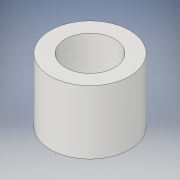
# Autodesk Inventor part: Spacer (Nylon), .313''OD, 0.25''
Saved by Autodesk Inventor 2018 (Build 220112000, 112)
## iProperties
Created: 2018-06-13
Part Number: Spacer (Nylon), .313''OD, 0.25''
Material: ABS Plastic
Document SubType Name: Modeling
Designer: s2sid
Density: 1.06 g/cm^3
Appearance: Smooth - White
Author: s2sid
Autodesk Inventor part; units mm, degrees
ref_plane "YZ Plane" through (0, 0, 0) normal (1, 0, 0) x (0, 1, 0)
ref_plane "XZ Plane" through (0, 0, 0) normal (0, 1, 0) x (-1, 0, 0)
ref_plane "XY Plane" through (0, 0, 0) normal (0, 0, 1) x (1, 0, 0)
sketch "Sketch1" plane through (0, 0, 0) normal (0, 1, 0) x (-1, 0, 0)
  circle A0 centre (0, 0) radius 2.4638
  circle A1 centre (0, 0) radius 3.9688
  dimension "d0" = 4.9276
  dimension "d1" = 7.9375
  constraints: 2 centre point, 2 coincident
  measures "d0" diameter of A0
  measures "d1" diameter of A1
extrude "Extrusion2" add sketch "Sketch1" along normal blind 6.35
body "Solid2"
